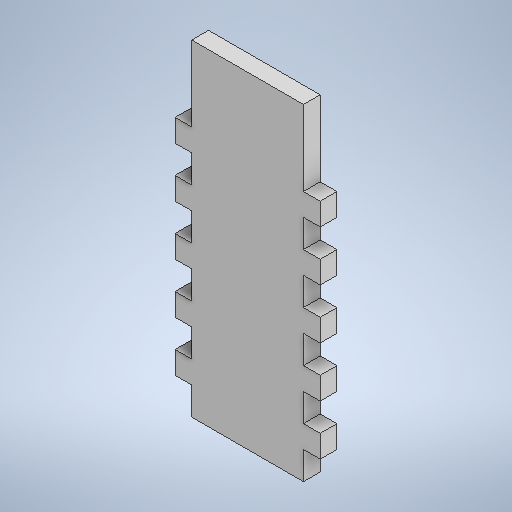
# Autodesk Inventor part: sort support wall 2
Saved by Autodesk Inventor 2025.3 (Build 293356000, 356)
## iProperties
Created: 2026-04-27
Part Number: sort support wall 2
Material: Generic
Document SubType Name: Modeling
Designer: kamal
Density: 1 g/cm^3
Appearance: Default
Author: kamal
Autodesk Inventor part; units mm, degrees
ref_plane "YZ Plane" through (0, 0, 0) normal (1, 0, 0) x (0, 1, 0)
ref_plane "XZ Plane" through (0, 0, 0) normal (0, 1, 0) x (-1, 0, 0)
ref_plane "XY Plane" through (0, 0, 0) normal (0, 0, 1) x (1, 0, 0)
sketch "Sketch1" plane through (0, 0, 0) normal (0, 0, 1) x (1, 0, 0)
  line L0 (0, 0) -> (-20, 0)
  line L1 (-20, 0) -> (-20, 10)
  line L2 (-20, 10) -> (-26, 10)
  line L3 (-26, 10) -> (-26, 18)
  line L4 (-26, 18) -> (-20, 18)
  line L5 (-20, 18) -> (-20, 28)
  line L6 (-20, 28) -> (-26, 28)
  line L7 (-26, 28) -> (-26, 36)
  line L8 (-26, 36) -> (-20, 36)
  line L9 (-20, 36) -> (-20, 46)
  line L10 (-20, 46) -> (-26, 46)
  line L11 (-26, 46) -> (-26, 54)
  line L12 (-26, 54) -> (-20, 54)
  line L13 (-20, 54) -> (-20, 64)
  line L14 (-20, 64) -> (-26, 64)
  line L15 (-26, 64) -> (-26, 72)
  line L16 (-26, 72) -> (-20, 72)
  line L17 (-20, 72) -> (-20, 82)
  line L18 (-20, 82) -> (-26, 82)
  line L19 (-26, 82) -> (-26, 90)
  line L20 (-26, 90) -> (-20, 90)
  line L21 (-20, 90) -> (-20, 117)
  line L22 (-20, 117) -> (0, 117)
  line L23 (0, 117) -> (0, 0) construction
  line L24 (0, 0) -> (20, 0)
  line L25 (20, 0) -> (20, 10)
  line L26 (20, 10) -> (26, 10)
  line L27 (26, 10) -> (26, 18)
  line L28 (26, 18) -> (20, 18)
  line L29 (20, 18) -> (20, 28)
  line L30 (26, 28) -> (26, 36)
  line L31 (26, 36) -> (20, 36)
  line L32 (20, 36) -> (20, 46)
  line L33 (20, 46) -> (26, 46)
  line L34 (26, 46) -> (26, 54)
  line L35 (26, 54) -> (20, 54)
  line L36 (20, 54) -> (20, 64)
  line L37 (20, 64) -> (26, 64)
  line L38 (26, 64) -> (26, 72)
  line L39 (26, 72) -> (20, 72)
  line L40 (20, 72) -> (20, 82)
  line L41 (20, 82) -> (26, 82)
  line L42 (26, 82) -> (26, 90)
  line L43 (26, 90) -> (20, 90)
  line L44 (20, 90) -> (20, 117)
  line L45 (20, 117) -> (0, 117)
  line L46 (20, 28) -> (26, 28)
  point P0 (-23, 90)
  dimension "d18" = 20
  dimension "d20" = 6
  dimension "d21" = 8
  dimension "d22" = 10
  dimension "d23" = 6
  dimension "d24" = 8
  dimension "d25" = 117
  dimension "d33" = 8
  dimension "d34" = 8
  dimension "d35" = 8
  dimension "d36" = 10
  dimension "d37" = 10
  dimension "d38" = 10
  dimension "d39" = 20
  dimension "d42" = 90
  constraints: 94 end point, 32 point on line, 22 symmetric about line, 11 perpendicular, 3 horizontal, 1 midpoint, 1 parallel
  measures "d18" distance of L0.start L0.end
  measures "d20" distance of L1.end L2.end
  measures "d21" distance of L2.end L3.end
  measures "d22" distance of L4.end L5.end
  measures "d23" distance of L5.end L6.end
  measures "d24" distance of L6.end L7.end
  measures "d25" distance between parallel lines of L0 L22
  measures "d33" distance of L10.end L11.end
  measures "d34" distance of L14.end L15.end
  measures "d35" distance of L18.end L19.end
  measures "d36" distance of L8.end L9.end
  measures "d37" distance of L12.end L13.end
  measures "d38" distance of L16.end L17.end
  measures "d39" distance from line of L22.end L17
  measures "d42" vertical distance of L0.end point (-23, 90)
extrude "Extrusion1" add sketch "Sketch1" along normal blind 6
body "Solid1"
